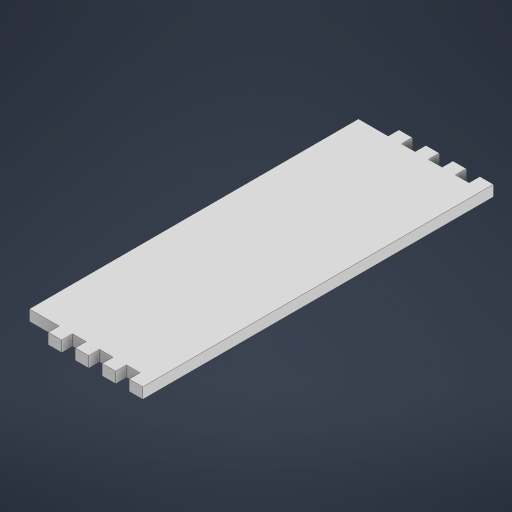
# Autodesk Inventor part: Angle_Zwischenebene
Saved by Autodesk Inventor 2023 (Build 270158030, 158C)
## iProperties
Created: 2022-06-23
Part Number: Angle_Zwischenebene
Material: Generic
Document SubType Name: Modeling
Designer: Simon
Density: 1 g/cm^3
Appearance: Default
Author: Simon
Autodesk Inventor part; units mm, degrees
ref_plane "YZ Plane" through (0, 0, 0) normal (1, 0, 0) x (0, 1, 0)
ref_plane "XZ Plane" through (0, 0, 0) normal (0, 1, 0) x (-1, 0, 0)
ref_plane "XY Plane" through (0, 0, 0) normal (0, 0, 1) x (1, 0, 0)
sketch "Sketch1" plane through (0, 0, 0) normal (0, 1, 0) x (-1, 0, 0)
  line L0 (11.02, 0) -> (0, 0)
  line L1 (-5, -122) -> (0, -122)
  line L2 (11.02, 0) -> (11.02, -122)
  line L3 (11.02, 0) -> (133.02, 0) construction
  line L4 (11.02, -122) -> (0, -122)
  line L5 (0, -126) -> (0, -122)
  line L6 (-5, -126) -> (-5, -122)
  line L7 (0, -126) -> (-5, -126)
  line L8 (-35, -122) -> (-30, -122)
  line L9 (-30, 0) -> (-35, 0)
  line L10 (0, -122) -> (-35, -122)
  line L11 (-35, -122) -> (-35, 0)
  line L12 (0, 0) -> (-35, 0)
  line L13 (-35, 0) -> (-35, 4)
  line L14 (-35, 4) -> (-30, 4)
  line L15 (-30, 0) -> (-30, 4)
  line L16 (-20, 0) -> (-20, 4)
  line L17 (-25, 4) -> (-20, 4)
  line L18 (-25, 0) -> (-25, 4)
  line L19 (-15, 0) -> (-15, 4)
  line L20 (-15, 4) -> (-10, 4)
  line L21 (-10, 0) -> (-10, 4)
  line L22 (0, 0) -> (0, 4)
  line L23 (-5, 4) -> (0, 4)
  line L24 (-5, 0) -> (-5, 4)
  line L25 (0, -126) -> (-5, -126)
  line L26 (-10, -126) -> (-10, -122)
  line L27 (-10, -126) -> (-15, -126)
  line L28 (-15, -126) -> (-15, -122)
  line L29 (-20, -126) -> (-20, -122)
  line L30 (-20, -126) -> (-25, -126)
  line L31 (-25, -126) -> (-25, -122)
  line L32 (-30, -126) -> (-30, -122)
  line L33 (-30, -126) -> (-35, -126)
  line L34 (-35, -126) -> (-35, -122)
  dimension "d0" = 90
  constraints: 70 end point, 7 horizontal, 3 perpendicular, 1 collinear, 5 other
  measures "d0" angle of L2 L3
extrude "Extrusion1" add sketch "Sketch1" along normal blind 4
body "Solid1"
